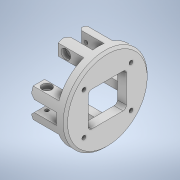
# Autodesk Inventor part: Motor_UR5_mount
Saved by Autodesk Inventor 2022 (Build 260153000, 153)
## iProperties
Created: 2021-08-03
Part Number: Motor_UR5_mount
Material: Generic
Document SubType Name: Modeling
Designer: exllu
Density: 1 g/cm^3
Appearance: Default
Author: exllu
Autodesk Inventor part; units mm, degrees
sketch "Sketch1" plane through (0, 0, 0) normal (1, 0, 0) x (0, 1, 0)
  circle A0 centre (0, 0) radius 15.75
  line L0 (0, 0) -> (0, 15.75)
  line L1 (0, 15.75) -> (-5, 15.75)
  line L2 (-5, 15.75) -> (5, 15.75)
  line L3 (5, 15.75) -> (5, -15.75)
  line L4 (5, -15.75) -> (-5, -15.75)
  line L5 (-5, -15.75) -> (-5, 15.75)
  line L6 (0, 0) -> (-15.75, 0)
  line L7 (-15.75, 0) -> (-15.75, -5)
  line L8 (-15.75, -5) -> (-15.75, 5)
  line L9 (-15.75, 5) -> (15.75, 5)
  line L10 (15.75, 5) -> (15.75, -5)
  line L11 (15.75, -5) -> (-15.75, -5)
  circle A1 centre (0, 0) radius 13.25
  point P0 (-5, -12.2704)
  point P1 (-12.2704, -5)
  point P2 (-14.9353, -5)
  point P3 (-5, -14.9353)
  point P4 (-12.2704, 5)
  point P5 (-5, 12.2704)
  point P6 (-5, 14.9353)
  point P7 (-14.9353, 5)
  point P8 (5, 12.2704)
  point P9 (12.2704, 5)
  point P10 (14.9353, 5)
  point P11 (5, 14.9353)
  point P12 (12.2704, -5)
  point P13 (5, -12.2704)
  point P14 (5, -14.9353)
  point P15 (14.9353, -5)
  dimension "d0" = 31.5
  dimension "d1" = 5
  dimension "d2" = 10
  dimension "d5" = 90
  dimension "d7" = 26.5
  constraints: 24 end point, 2 coincident, 2 horizontal, 2 parallel, 2 perpendicular, 1 centre point, 1 vertical, 16 other
  measures "d1" distance of L0.end L1.end
  measures "d2" distance of L3.end L4.end
  measures "d7" diameter of A1
sketch "Sketch2" plane through (0, 0, 0) normal (1, 0, 0) x (0, 1, 0)
  circle A0 centre (0, 0) radius 37.5
  line L0 (0, 37.5) -> (-5, 37.5)
  line L1 (0, 37.5) -> (5, 37.5) construction
  line L2 (-5, 37.5) -> (5, 37.5)
  line L3 (5, 37.5) -> (5, -37.5)
  line L4 (5, -37.5) -> (-5, -37.5)
  line L5 (-5, -37.5) -> (-5, 37.5)
  circle A1 centre (0, 0) radius 37.5
  line L6 (-37.5, 0) -> (-37.5, -5)
  line L7 (-37.5, 0) -> (-37.5, 5) construction
  line L8 (-37.5, -5) -> (-37.5, 5)
  line L9 (-37.5, 5) -> (37.5, 5)
  line L10 (37.5, 5) -> (37.5, -5)
  line L11 (37.5, -5) -> (-37.5, -5)
  circle A2 centre (0, 0) radius 32.5
  line L12 (0, 0) -> (24, 0)
  line L13 (24, 0) -> (24, 21.9146)
  line L14 (24, 21.9146) -> (24, -21.9146)
  line L15 (-21.9146, 24) -> (21.9146, 24)
  line L16 (-24, -21.9146) -> (-24, 21.9146)
  line L17 (21.9146, -24) -> (-21.9146, -24)
  line L18 (-24, 5) -> (-29, 5)
  line L19 (-29, 5) -> (-29, 14.6714)
  line L20 (-29, 14.6714) -> (-29, -14.6714)
  line L21 (-29, -5) -> (-29, -8)
  line L22 (-29, -8) -> (-26, -8)
  line L23 (-26, -8) -> (-26, -5)
  line L24 (-29, -5) -> (-26, -5)
  line L25 (-29, 5) -> (-26, 5)
  line L26 (-26, 5) -> (-26, 8)
  line L27 (-26, 8) -> (-29, 8)
  line L28 (-29, 8) -> (-29, 5)
  line L29 (-32.1131, -5) -> (-26, -5)
  line L30 (-26, -5) -> (-26, -22.6317)
  line L31 (-26, -22.6317) -> (-26, 21.6916)
  point P0 (-32.1131, 5)
  point P1 (-5, 32.1131)
  point P2 (-5, 37.1652)
  point P3 (-37.1652, 5)
  point P4 (-5, -32.1131)
  point P5 (-37.1652, -5)
  point P6 (-5, -37.1652)
  point P7 (32.1131, -5)
  point P8 (5, -32.1131)
  point P9 (5, -37.1652)
  point P10 (37.1652, -5)
  point P11 (5, 32.1131)
  point P12 (32.1131, 5)
  point P13 (37.1652, 5)
  point P14 (5, 37.1652)
  point P15 (-5, 24)
  point P16 (5, 24)
  point P17 (24, 5)
  point P18 (24, -5)
  point P19 (-5, -24)
  point P20 (5, -24)
  point P21 (-26, 19.5)
  point P22 (-26, -19.5)
  dimension "d10" = 75
  dimension "d11" = 5
  dimension "d12" = 180
  dimension "d15" = 90
  dimension "d17" = 65
  dimension "d42" = 24
  dimension "d45" = 360
  dimension "d54" = 5
  dimension "d55" = 3
  dimension "d56" = 3
  dimension "d57" = 3
  dimension "d58" = 3
  constraints: 64 end point, 11 point on line, 6 perpendicular, 5 horizontal, 5 point on circle, 4 parallel, 3 collinear, 2 coincident, 1 centre point, 1 horizontal alignment, 1 vertical, 33 other
  measures "d11" distance of L0.start L0.end
  measures "d12" angle of L0 L1
  measures "d17" diameter of A2
  measures "d42" distance of L12.start L12.end
  measures "d54" distance of L18.start L18.end
  measures "d55" distance of L21.start L21.end
  measures "d56" distance of L21.end L22.end
  measures "d57" distance of L27.end L26.end
  measures "d58" distance of L26.end L25.end
extrude "Extrusion2" add sketch "Sketch2" along normal blind 20 contours L9 A2 L3 A0 | A0 L3 A2 L11 | L5 A2 L9 A0 | A0 L11 A2 L5
sketch "Sketch3" plane through (20, 0, 0) normal (1, 0, 0) x (0, 0, -1)
  circle A0 centre (0, 0) radius 37.5
  constraints: 1 centre point, 1 coincident
extrude "Extrusion3" add sketch "Sketch3" along normal blind 8
sketch "Sketch5" plane through (20, 0, 0) normal (-1, 0, 0) x (0, 0, 1)
  line L0 (0, 0) -> (17.6777, 17.6777)
  line L1 (0, 0) -> (25, 0) construction
  circle A0 centre (17.6777, 17.6777) radius 5
  dimension "d39" = 25
  dimension "d40" = 45
  dimension "d41" = 10
  constraints: 4 end point, 1 centre point, 1 coincident, 1 equal length, 1 horizontal
  measures "d39" distance of L0.start L0.end
  measures "d40" angle of L1 L0
  measures "d41" diameter of A0
extrude "Extrusion6" add sketch "Sketch2" along normal blind 20 contours L9 L13 A2 | A2 L14 L11 | A2 L15 L3 | L3 L17 A2 | L5 L15 A2 | A2 L17 L5
sketch "Sketch7" plane through (20, 0, 0) normal (-1, 0, 0) x (0, 0, 1)
  circle A0 centre (-11, -22) radius 1.3 projected
  circle A1 centre (-11, -22) radius 2.25
  circle A2 centre (-11, 18) radius 1.3 projected
  circle A3 centre (-11, 18) radius 2.25
  circle A4 centre (11, 18) radius 1.3 projected
  circle A5 centre (11, 18) radius 2.25
  circle A6 centre (11, -22) radius 1.3 projected
  circle A7 centre (11, -22) radius 2.25
  circle A8 centre (-11, 18) radius 4
  circle A9 centre (11, 18) radius 4
  circle A10 centre (-11, -22) radius 4
  circle A11 centre (11, -22) radius 1.3 projected
  circle A12 centre (11, -22) radius 4
  line L0 (-5, -32.1131) -> (-5, -37.1652) projected
  arc A13 (-24, -21.9146) -> (-5, -32.1131) centre (0, 0) ccw projected
  arc A14 (5, -32.1131) -> (24, -21.9146) centre (0, 0) ccw projected
  dimension "d59" = 4.5
  dimension "d60" = 4.5
  dimension "d61" = 4.5
  dimension "d62" = 4.5
  dimension "d63" = 8
  dimension "d64" = 8
  dimension "d65" = 8
  dimension "d66" = 8
  constraints: 8 centre point, 8 coincident
  measures "d59" diameter of A1
  measures "d60" diameter of A3
  measures "d61" diameter of A5
  measures "d62" diameter of A7
  measures "d63" diameter of A8
  measures "d64" diameter of A9
  measures "d65" diameter of A10
  measures "d66" diameter of A12
extrude "Extrusion7" add sketch "Sketch2" along normal blind 20 contours A2 L19 L9 | L11 L20 A2 | L19 L27 L26 L9 | A2 L31 L27 L19 | L11 L23 L22 L20 | L20 L22 L30 A2
sketch "Sketch8" plane through (0, 0, 0) normal (-1, 0, 0) x (0, 0, 1)
  line L0 (-5, -26) -> (-5, -37.1652) projected
  line L1 (-5, -26) -> (-5, -28)
  line L2 (-5, -28) -> (-13, -28)
  line L3 (-13, -28) -> (-13, -35.1746)
  arc A0 (-37.1652, -5) -> (-5, -37.1652) centre (0, 0) ccw projected
  line L4 (-13, -28) -> (-24.9449, -28)
  dimension "d69" = 2
  dimension "d70" = 8
  constraints: 8 end point, 2 point on circle, 1 horizontal, 1 perpendicular, 1 point on line, 1 vertical
  measures "d69" distance of L0.start L1.end
  measures "d70" distance of L1.end L2.end
extrude "Extrusion8" cut sketch "Sketch8" against normal blind 10 contours L3 A0 L4
ref_plane "Work Plane1" through (20, -37.1652, 0) normal (0, 0, -1) x (-1, 0, 0)
mirror "Mirror1" about plane through (20, -37.1652, 0) normal (0, 0, -1) of "Extrusion8"
sketch "Sketch9" plane through (0, 0, 0) normal (-1, 0, 0) x (0, 0, 1)
  line L0 (-5, 37.1652) -> (-5, 24) projected
  line L1 (-5, 24) -> (-5, 27)
  line L2 (-5, 27) -> (-13, 27)
  line L3 (-13, 27) -> (-13, 35.1746)
  circle A0 centre (0, 0) radius 37.5 projected
  line L4 (-13, 27) -> (-27.1603, 27)
  point P0 (-26.024, 27)
  dimension "d73" = 3
  dimension "d74" = 8
  constraints: 8 end point, 2 point on line, 1 horizontal, 1 perpendicular, 1 point on circle
  measures "d73" distance of L0.end L1.end
  measures "d74" distance of L1.end L2.end
extrude "Extrusion9" cut sketch "Sketch9" against normal blind 15 contours L3 L4 A0
mirror "Mirror2" about plane through (20, -37.1652, 0) normal (0, 0, -1) of "Extrusion9"
sketch "Sketch10" plane through (20, -37.1652, 0) normal (0, 0, -1) x (-1, 0, 0)
  line L0 (0, 42.1652) -> (0, 32.1652) projected
  line L1 (0, 37.1652) -> (8.9851, 37.1652)
  point P0 (20, 37.1652)
  constraints: 2 end point, 1 horizontal, 1 midpoint
pattern_circular "Circular Pattern1" count 2 over 90 about axis through (20, 0, 0) along (-1, 0, 0) of "Extrusion9", "Mirror2"
mirror "Mirror3" about plane through (20, -37.1652, 0) normal (0, 0, -1) of "Extrusion9", "Mirror2", "Circular Pattern1"
sketch "Sketch11" plane through (0, 0, 0) normal (-1, 0, 0) x (0, 0, 1)
  circle A0 centre (0, 0) radius 37.5
  line L0 (-5, 37.1652) -> (-5, 24) projected
  line L1 (-5, 24) -> (-5, 37.1652)
  line L2 (-13, 35.1746) -> (-13, 27) projected
  line L3 (-13, 27) -> (-13, 35.1746)
  line L4 (-13, 27) -> (-13, 24)
  line L5 (-5, 24) -> (-21.9146, 24) projected
  line L6 (-5, 24) -> (-13, 24)
  constraints: 8 end point, 3 collinear, 1 centre point, 1 coincident, 1 point on line, 1 vertical
extrude "Extrusion10" add sketch "Sketch11" along normal blind 10 contours L0 L5 L4 L2 A0 picked at (-8.571, 29.2327)
mirror "Mirror4" about plane through (20, -37.1652, 0) normal (0, 0, -1) of "Extrusion10"
pattern_circular "Circular Pattern2" count 2 over 90 about axis through (20, 0, 0) along (-1, 0, 0) of "Extrusion10", "Mirror4"
mirror "Mirror5" about plane through (20, -37.1652, 0) normal (0, 0, -1) of "Extrusion10", "Mirror4", "Circular Pattern2"
sketch "Sketch12" plane through (0, 0, 0) normal (-1, 0, 0) x (0, 0, 1)
  line L0 (-35.1746, 13) -> (-24, 13) projected
  line L1 (-24, 13) -> (-40.3867, 13)
  line L2 (-40.3867, 13) -> (-13, 13)
  line L3 (-13, 13) -> (-13, 36.1973)
  line L4 (-13, 36.1973) -> (-40.3867, 36.1973)
  line L5 (-40.3867, 36.1973) -> (-40.3867, 13)
  point P0 (0, 0)
  constraints: 10 end point, 2 horizontal, 2 parallel, 1 perpendicular
extrude "Extrusion11" cut sketch "Sketch12" against normal blind 15
mirror "Mirror6" about plane through (20, -37.1652, 0) normal (0, 0, -1) of "Extrusion11"
sketch "Sketch13" plane through (0, 0, 0) normal (-1, 0, 0) x (0, 0, 1)
  line L0 (-5, -26) -> (-5, -32.1131) projected
  line L1 (-5, -26) -> (-5, -38.6287)
  line L2 (-19.5, -26) -> (-5, -26) projected
  line L3 (-5, -26) -> (-13, -26)
  line L4 (-13, -28) -> (-13, -35.1746) projected
  line L5 (-13, -26) -> (-13, -35.1746)
  circle A0 centre (0, 0) radius 37.5
  point P0 (-5, -37.1652)
  dimension "d87" = 8
  constraints: 6 end point, 1 centre point, 1 coincident, 1 point on line, 1 vertical
  measures "d87" distance of L0.start L3.end
extrude "Extrusion12" add sketch "Sketch13" along normal blind 10 contours L0 L1 A0 L4 L5 L2 picked at (-9.4615, -32.0489)
mirror "Mirror7" about plane through (20, -37.1652, 0) normal (0, 0, -1) of "Extrusion12"
sketch "Sketch14" plane through (0, 0, 0) normal (-1, 0, 0) x (0, 0, 1)
  line L0 (-24, -13) -> (-24, -5) projected
  line L1 (-24, -13) -> (-44.4071, -13)
  line L2 (-13, -26) -> (-13, -35.1746) projected
  line L3 (-44.4071, -13) -> (-13, -13)
  line L4 (-13, -13) -> (-13, -30.5873)
  line L5 (-44.4071, -30.5873) -> (-44.4071, -13)
  line L6 (-13, -13) -> (-44.4071, -13)
  line L7 (-44.4071, -13) -> (-44.4071, -39.7586)
  line L8 (-44.4071, -39.7586) -> (-13, -39.7586)
  line L9 (-13, -39.7586) -> (-13, -13)
  point P0 (0, 0)
  constraints: 16 end point, 3 horizontal, 3 parallel, 2 perpendicular, 1 midpoint
extrude "Extrusion13" cut sketch "Sketch14" against normal blind 15
mirror "Mirror8" about plane through (20, -37.1652, 0) normal (0, 0, -1) of "Extrusion13"
sketch "Sketch15" plane through (15, 24, -13) normal (0, 0, -1) x (-1, 0, 0)
  line L0 (0, 0) -> (11, 0)
  line L1 (11, 0) -> (11, 6)
  line L2 (25, 13.1652) -> (-5, 13.1652) projected
  circle A0 centre (11, 6) radius 1.65
  point P0 (15, -24)
  dimension "d92" = 11
  dimension "d93" = 6
  dimension "d94" = 3.3
  constraints: 4 end point, 1 centre point, 1 coincident, 1 horizontal, 1 perpendicular
  measures "d92" distance of L0.start L0.end
  measures "d93" distance of L0.end L1.end
  measures "d94" diameter of A0
extrude "Extrusion14" cut sketch "Sketch15" against normal blind 30
pattern_circular "Circular Pattern3" count 2 over 90 about axis through (20, 0, 0) along (-1, 0, 0) of "Extrusion14"
pattern_circular "Circular Pattern4" count 2 over 90 about axis through (20, 0, 0) along (1, 0, 0) of "Extrusion14"
sketch "Sketch16" plane through (15, -35.1746, -13) normal (0, 0, -1) x (-1, 0, 0)
  line L0 (0, 22.1746) -> (0, 0) projected
  line L1 (0, 0) -> (11, 0)
  line L2 (25, 0) -> (0, 0) projected
  line L3 (11, 0) -> (11, 4)
  circle A0 centre (11, 4) radius 1.65
  point P0 (15, 35.1746)
  dimension "d103" = 11
  dimension "d104" = 4
  dimension "d105" = 3.3
  constraints: 4 end point, 1 centre point, 1 coincident, 1 point on line, 1 vertical
  measures "d103" distance of L0.end L1.end
  measures "d104" distance of L1.end L3.end
  measures "d105" diameter of A0
extrude "Extrusion15" cut sketch "Sketch16" against normal blind 30
chamfer "Chamfer1" distance 2 angle 45 1 edges at (28, 0, 37.5)
sketch "Sketch18" plane through (15, 0, 0) normal (-1, 0, 0) x (0, 0, 1)
  line L0 (-13, 24) -> (-5, 24) projected
  line L1 (-13, 24) -> (-13, 8.8948)
  line L2 (-35.1746, 13) -> (-27, 13) projected
  line L3 (-24, 13) -> (-11.2178, 13)
  line L4 (-13, 13) -> (-36.9172, 13)
  line L5 (-36.9172, 13) -> (-36.9172, 36.9183)
  line L6 (-36.9172, 36.9183) -> (-13, 36.9183)
  line L7 (-13, 36.9183) -> (-13, 13)
  line L8 (0, 0) -> (0, 5.9955)
  line L9 (0, 0) -> (-9, 0)
  line L10 (-13, -24) -> (-5, -24)
  line L11 (-13, -24) -> (-13, -8.8948)
  line L12 (-35.1746, -13) -> (-24, -13)
  line L13 (-24, -13) -> (-11.2178, -13)
  line L14 (-13, -13) -> (-36.9172, -13)
  line L15 (-36.9172, -13) -> (-36.9172, -36.9183)
  line L16 (-36.9172, -36.9183) -> (-13, -36.9183)
  line L17 (-13, -36.9183) -> (-13, -13)
  line L18 (13, 24) -> (5, 24)
  line L19 (13, 24) -> (13, 8.8948)
  line L20 (35.1746, 13) -> (24, 13)
  line L21 (24, 13) -> (11.2178, 13)
  line L22 (13, 13) -> (36.9172, 13)
  line L23 (36.9172, 13) -> (36.9172, 36.9183)
  line L24 (36.9172, 36.9183) -> (13, 36.9183)
  line L25 (13, 36.9183) -> (13, 13)
  line L26 (0, 0) -> (9, 0)
  line L27 (13, -24) -> (5, -24)
  line L28 (13, -24) -> (13, -8.8948)
  line L29 (35.1746, -13) -> (24, -13)
  line L30 (24, -13) -> (11.2178, -13)
  line L31 (13, -13) -> (36.9172, -13)
  line L32 (36.9172, -13) -> (36.9172, -36.9183)
  line L33 (36.9172, -36.9183) -> (13, -36.9183)
  line L34 (13, -36.9183) -> (13, -13)
  constraints: 66 end point, 31 symmetric about line, 8 point on line, 2 horizontal, 2 parallel, 2 perpendicular, 2 vertical
extrude "Extrusion17" cut sketch "Sketch18" against normal blind 5
sketch "Sketch19" plane through (20, 0, 0) normal (-1, 0, 0) x (0, 0, 1)
  circle A0 centre (-11, 18) radius 1.3 projected
  line L0 (0, 0) -> (-11, 0)
  line L1 (-11, 0) -> (-11, 18)
  line L2 (-11, 18) -> (0, 18)
  line L3 (0, 18) -> (0, 0)
  line L4 (-11, 18) -> (-21, 18)
  line L5 (-21, 18) -> (-21, 18.5)
  circle A1 centre (-21, 18.5) radius 3.25
  circle A2 centre (21, 18.5) radius 3.25
  circle A3 centre (-21, -18.5) radius 3.25
  circle A4 centre (21, -18.5) radius 3.25
  point P0 (-9.7, 18)
  point P1 (-11, 16.7)
  point P2 (-12.3, 18)
  dimension "d122" = 10
  dimension "d123" = 0.5
  dimension "d124" = 6.5
  constraints: 12 end point, 4 centre point, 3 symmetric about line, 2 horizontal, 2 parallel, 2 perpendicular, 1 coincident, 3 other
  measures "d122" distance of L1.end L4.end
  measures "d123" distance of L4.end L5.end
  measures "d124" diameter of A1
extrude "Extrusion18" cut sketch "Sketch19" against normal blind 3 contours A1 | A2 | A3 | A4
sketch "Sketch20" plane through (20, 0, 0) normal (-1, 0, 0) x (0, 0, 1)
  circle A0 centre (-21, 18.5) radius 3.25 projected
  circle A1 centre (-21, 18.5) radius 1.7
  circle A2 centre (21, 18.5) radius 3.25 projected
  circle A3 centre (21, 18.5) radius 1.7
  circle A4 centre (21, -18.5) radius 3.25 projected
  circle A5 centre (21, -18.5) radius 1.7
  circle A6 centre (-21, -18.5) radius 3.25 projected
  circle A7 centre (-21, -18.5) radius 1.7
  point P0 (0, 0)
  dimension "d127" = 3.4
  dimension "d128" = 3.4
  dimension "d129" = 3.4
  dimension "d130" = 3.4
  constraints: 4 centre point, 4 coincident
  measures "d127" diameter of A1
  measures "d128" diameter of A3
  measures "d129" diameter of A5
  measures "d130" diameter of A7
extrude "Extrusion19" cut sketch "Sketch20" against normal blind 10 contours A1 | A3 | A5 | A7
ref_plane "Work Plane2" through (20, 0, -24) normal (0, 1, 0) x (1, 0, 0)
sketch "Sketch21" plane through (20, 0, 0) normal (-1, 0, 0) x (0, 0, 1)
  line L0 (-14.7479, -24.8335) -> (17.8889, -24.8335)
  line L1 (17.8889, -24.8335) -> (17.8889, -39.2624)
  line L2 (17.8889, -39.2624) -> (-14.7479, -39.2624)
  line L3 (-14.7479, -39.2624) -> (-14.7479, -24.8335)
  point P0 (0, 0)
  constraints: 8 end point, 2 parallel, 1 horizontal, 1 perpendicular
extrude "Extrusion20" cut sketch "Sketch21" along normal blind 60
sketch "Sketch22" plane through (20, 0, 0) normal (-1, 0, 0) x (0, 0, 1)
  line L0 (-5, 24) -> (5, 24)
  line L1 (5, 24) -> (5, -67.8209)
  line L2 (5, -67.8209) -> (-5, -67.8209)
  line L3 (-5, -67.8209) -> (-5, 24)
  line L4 (-13, 26) -> (-5, 26)
  line L5 (-5, 26) -> (-5, -42.5951)
  line L6 (-5, -42.5951) -> (-13, -42.5951)
  line L7 (-13, -42.5951) -> (-13, 26)
  line L8 (13, 26) -> (11, 24) projected
  line L9 (13, 26) -> (5, 26)
  line L10 (5, 26) -> (5, -42.1761)
  line L11 (5, -42.1761) -> (13, -42.1761)
  line L12 (13, -42.1761) -> (13, 26)
  arc A0 (-35.1746, -13) -> (35.1746, -13) centre (0, 0) ccw projected
  line L13 (-5, -37.1652) -> (-13, -37.1652)
  line L14 (-13, -37.1652) -> (-13, -24.0002)
  line L15 (-13, -24.0002) -> (-5, -24.0002)
  line L16 (-5, -24.0002) -> (-5, -37.1652)
  line L17 (5, -37.1652) -> (13, -37.1652)
  line L18 (13, -37.1652) -> (13, -24.0002)
  line L19 (13, -24.0002) -> (5, -24.0002)
  line L20 (5, -24.0002) -> (5, -37.1652)
  point P0 (-13, -35.1746)
  point P1 (-5, -37.1652)
  point P2 (5, -37.1652)
  point P3 (13, -35.1746)
  dimension "d141" = 13.165
  dimension "d142" = 8
  dimension "d143" = 13.165
  constraints: 40 end point, 10 parallel, 5 horizontal, 5 perpendicular, 5 point on line, 2 point on circle
  measures "d141" distance of L13.end L14.end
  measures "d142" distance of L19.end L18.end
  measures "d143" distance of L18.end L17.end
extrude "Extrusion21" add sketch "Sketch22" along normal blind 30 contours L3 A0 L7 L15 | L19 L12 A0 L1
mirror "Mirror10" about plane through (20, 0, -24) normal (0, 1, 0) of "Extrusion14"
sketch "Sketch23" plane through (-10, 35.1746, 13) normal (0, 0, 1) x (1, 0, 0)
  circle A0 centre (14, -5.1746) radius 1.65 projected
  circle A1 centre (14, -5.1746) radius 4.25
  point P0 (10, -35.1746)
  dimension "d149" = 8.5
  constraints: 1 centre point, 1 coincident
  measures "d149" diameter of A1
extrude "Extrusion22" cut sketch "Sketch23" against normal blind 4
sketch "Sketch24" plane through (-10, -35.1746, 13) normal (0, 0, 1) x (1, 0, 0)
  circle A0 centre (14, 5.1746) radius 1.65 projected
  circle A1 centre (14, 5.1746) radius 4.25
  point P0 (10, 35.1746)
  dimension "d152" = 8.5
  constraints: 1 centre point, 1 coincident
  measures "d152" diameter of A1
extrude "Extrusion23" cut sketch "Sketch24" against normal blind 4
ref_plane "Work Plane3" through (-10, -35.1746, 0) normal (0, 0, 1) x (1, 0, 0)
mirror "Mirror11" about plane through (-10, -35.1746, 0) normal (0, 0, 1) of "Extrusion22", "Extrusion23"
sketch "Sketch25" plane through (20, -13, 24) normal (0, -1, 0) x (1, 0, 0)
  circle A0 centre (-16, 6) radius 1.65 projected
  circle A1 centre (-16, 6) radius 4.25
  circle A2 centre (-16, -54) radius 1.65 projected
  circle A3 centre (-16, -54) radius 4.25
  point P0 (-20, -24)
  dimension "d158" = 8.5
  dimension "d159" = 8.5
  constraints: 2 centre point, 2 coincident
  measures "d158" diameter of A1
  measures "d159" diameter of A3
extrude "Extrusion24" cut sketch "Sketch25" against normal blind 4 contours A0 | A1 | A2 | A3
ref_plane "Work Plane4" through (20, 0, 24) normal (0, -1, 0) x (1, 0, 0)
mirror "Mirror12" about plane through (20, 0, 24) normal (0, -1, 0) of "Extrusion24"
chamfer "Chamfer7" distance 1 angle 45 11 edges at (-5, 13, -24) (17.5, 24, -13) (-5, 24, -13) (-5, 24, 13) (17.5, 13, 24) (2.5, 13, 24) (-5, -13, 24) (5, -24.0002, 13) (5, -24.0002, -13) (17.5, -13, -24) (-5, -13, -24)
sketch "Sketch26" plane through (-10, 5, 24) normal (-1, 0, 0) x (0, 0, 1)
  circle A0 centre (-24, -5) radius 46.672
  constraints: 1 centre point, 1 coincident
extrude "Extrusion25" cut sketch "Sketch26" against normal blind 7
chamfer "Chamfer8" distance 3 angle 45 8 edges at (-3, 30.5826, 5) (-3, -30.5827, 5) (-3, 30.5826, -5) (-3, -30.5827, -5) (-3, 5, -30.5826) (-3, 5, 30.5826) (-3, -5, -30.5826) (-3, -5, 30.5826)
sketch "Sketch27" plane through (20, 0, 0) normal (-1, 0, 0) x (0, 0, 1)
  circle A0 centre (-21, 18.5) radius 1.7 projected
  line L0 (-21, 18.5) -> (-13.75, 18.5)
  line L1 (-13.75, 18.5) -> (-13.75, 12.14)
  line L2 (-21, 18.5) -> (5, 18.5)
  line L3 (5, 18.5) -> (5, 4.14)
  line L4 (5, 18.5) -> (5, -8.56)
  circle A1 centre (-13.75, 12.14) radius 3.25
  circle A2 centre (5, 4.14) radius 3.25
  circle A3 centre (5, -8.56) radius 3.25
  point P0 (0, 0)
  dimension "d170" = 7.25
  dimension "d171" = 6.36
  dimension "d172" = 26
  dimension "d173" = 14.36
  dimension "d174" = 27.06
  dimension "d175" = 6.5
  dimension "d176" = 6.5
  dimension "d177" = 6.5
  constraints: 10 end point, 3 centre point, 3 coincident, 2 horizontal, 2 perpendicular, 1 vertical
  measures "d170" distance of L0.start L0.end
  measures "d171" distance of L0.end L1.end
  measures "d172" distance of L0.start L2.end
  measures "d173" distance of L2.end L3.end
  measures "d174" distance of L2.end L4.end
  measures "d175" diameter of A1
  measures "d176" diameter of A2
  measures "d177" diameter of A3
extrude "Extrusion26" cut sketch "Sketch27" against normal blind 10 contours A2 L4 L3 | L3 L4 A2 | A1 | A3
sketch "Sketch28" plane through (20, 0, 0) normal (-1, 0, 0) x (0, 0, 1)
  circle A0 centre (-13.75, 12.14) radius 3.25 projected
  line L0 (-13.75, 12.14) -> (0, 12.14)
  line L1 (-13.75, 12.14) -> (-17, 12.14)
  line L2 (-17, 12.14) -> (-17, 15.39)
  line L3 (-17, 15.39) -> (-13.75, 15.39)
  line L4 (-13.75, 15.39) -> (-13.75, 12.14)
  line L5 (-17, 15.39) -> (17, 15.39)
  line L6 (17, 15.39) -> (17, -15.39)
  line L7 (17, -15.39) -> (-17, -15.39)
  line L8 (-17, -15.39) -> (-17, 15.39)
  point P0 (0, 0)
  dimension "d180" = 13.75
  dimension "d181" = 34
  dimension "d182" = 30.78
  dimension "d183" = 90
  constraints: 18 end point, 4 perpendicular, 2 horizontal, 2 parallel, 1 point on line
  measures "d180" distance of L0.start L0.end
  measures "d181" distance of L2.end L5.end
  measures "d182" distance of L5.end L6.end
  measures "d183" angle of L5 L6
extrude "Extrusion27" cut sketch "Sketch28" against normal blind 10
fillet "Fillet1" radius 3 4 edges at (24, 15.39, -17) (24, 15.39, 17) (24, -15.39, 17) (24, -15.39, -17)
body "Solid2"
